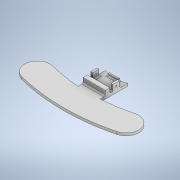
# Autodesk Inventor part: paddle
Saved by Autodesk Inventor 2020.3 (Build 243373010, 373A)
## iProperties
Created: 2020-09-18
Part Number: paddle
Material: Generic
Document SubType Name: Modeling
Designer: joesp
Density: 1 g/cm^3
Appearance: Default
Author: joesp
Autodesk Inventor part; units mm, degrees
ref_plane "YZ Plane" through (0, 0, 0) normal (1, 0, 0) x (0, 1, 0)
ref_plane "XZ Plane" through (0, 0, 0) normal (0, 1, 0) x (-1, 0, 0)
ref_plane "XY Plane" through (0, 0, 0) normal (0, 0, 1) x (1, 0, 0)
sketch "Sketch1" plane through (0, 0, 0) normal (0, 1, 0) x (-1, 0, 0)
  arc A0 (92.5, 31.0634) -> (-57.5, 31.0634) centre (17.5, -259.4104) ccw
  arc A1 (82.5, -7.6665) -> (92.5, 31.0634) centre (87.5, 11.6984) ccw
  arc A2 (-57.5, 31.0634) -> (-47.5, -7.6665) centre (-52.5, 11.6984) ccw
  arc A3 (82.5, -7.6665) -> (-47.5, -7.6665) centre (17.5, -259.4104) ccw
  line L0 (35, 0) -> (0, 0)
  line L1 (0, 0) -> (0, -50)
  line L2 (0, -50) -> (35, -50)
  line L3 (35, -50) -> (35, 0)
  point P0 (40, -0.7704)
  dimension "d0" = 140
  dimension "d1" = 20
  dimension "d2" = 52.5
  dimension "d4" = 300
  dimension "d5" = 50
  dimension "d8" = 35
  dimension "d9" = 52.5
  constraints: 10 point on circle, 8 end point, 4 centre point, 4 tangent, 2 coincident, 2 horizontal alignment, 2 perpendicular, 1 parallel
  measures "d0" distance of A2.centre A1.centre
  measures "d1" radius of A1
  measures "d2" horizontal distance of A1.centre L0.start
  measures "d4" radius of A0
  measures "d5" distance of L2.end L0.start
  measures "d8" distance of L1.end L2.end
  measures "d9" horizontal distance of A2.centre point (0, 0)
extrude "Extrusion1" add sketch "Sketch1" along normal blind 4
sketch "Sketch2" plane through (0, 4, 0) normal (0, 1, 0) x (1, 0, 0)
  line L0 (0, 30) -> (-3, 30)
  line L1 (-3, 30) -> (-3, 20)
  line L2 (-3, 20) -> (0, 20)
  line L3 (0, 20) -> (0, 30)
  line L4 (-35, 30) -> (-32, 30)
  line L5 (-32, 30) -> (-32, 20)
  line L6 (-32, 20) -> (-35, 20)
  line L7 (-35, 20) -> (-35, 30)
  line L8 (0, 0) -> (0, 50) projected
  line L9 (-35, 50) -> (-35, 0) projected
  point P0 (-35, 25)
  dimension "d10" = 3
  dimension "d11" = 3
  dimension "d12" = 10
  constraints: 16 end point, 4 parallel, 2 collinear, 2 horizontal, 2 midpoint, 2 perpendicular, 2 point on line
  measures "d10" distance of L0.start L0.end
  measures "d11" distance of L4.start L4.end
  measures "d12" distance of L4.end L5.end
extrude "Extrusion2" add sketch "Sketch2" along normal blind 10
sketch "Sketch3" plane through (0, 4, 0) normal (0, 1, 0) x (1, 0, 0)
  line L0 (-35, 15) -> (0, 15)
  line L1 (0, 15) -> (0, 8)
  line L2 (0, 8) -> (-35, 8)
  line L3 (-35, 8) -> (-35, 15)
  line L4 (0, 0) -> (0, 20) projected
  line L5 (-35, 20) -> (-35, 0) projected
  line L6 (-35, 50) -> (-35, 0) projected
  point P0 (-35, 25)
  dimension "d15" = 7
  dimension "d16" = 10
  constraints: 8 end point, 2 parallel, 2 point on line, 1 horizontal, 1 midpoint, 1 perpendicular
  measures "d15" distance of L2.end L0.start
  measures "d16" distance from line of L0 point (-35, 25)
extrude "Extrusion3" add sketch "Sketch3" along normal blind 8
sketch "Sketch4" plane through (0, 0, 0) normal (1, 0, 0) x (0, 0, -1)
  circle A0 centre (25, 9) radius 1.375
  line L0 (30, 4) -> (30, 14) projected
  line L1 (20, 14) -> (30, 14) projected
  point P0 (0, 0)
  point P1 (30, 9)
  point P2 (25, 14)
  dimension "d19" = 2.75
  constraints: 2 midpoint, 1 centre point, 1 horizontal alignment, 1 vertical alignment
  measures "d19" diameter of A0
extrude "Extrusion4" cut sketch "Sketch4" against normal through all
sketch "Sketch5" plane through (0, 4, 0) normal (0, 1, 0) x (1, 0, 0)
  line L0 (-25, 37.5) -> (-10, 37.5)
  line L1 (-10, 37.5) -> (-10, 41.5)
  line L2 (-10, 41.5) -> (-25, 41.5)
  line L3 (-25, 41.5) -> (-25, 37.5)
  line L4 (0, 20) -> (0, 30) projected
  line L5 (-35, 50) -> (-35, 30) projected
  line L6 (0, 30) -> (0, 50) projected
  point P0 (0, 0)
  point P1 (-10, 39.5)
  point P2 (0, 25)
  dimension "d22" = 4
  dimension "d23" = 15
  dimension "d26" = 14.5
  dimension "d27" = 10
  dimension "d28" = 10
  constraints: 8 end point, 2 midpoint, 2 parallel, 1 horizontal, 1 perpendicular
  measures "d22" distance of L2.end L0.start
  measures "d23" distance of L0.start L0.end
  measures "d26" vertical distance of point (0, 25) point (-10, 39.5)
  measures "d27" distance between parallel lines of L5 L3
  measures "d28" distance between parallel lines of L6 L1
extrude "Extrusion5" add sketch "Sketch5" along normal blind 3.625
chamfer "Chamfer1" distance 2 angle 45 12 edges at (-17.5, 4, -15) (-32, 4, -25) (-33.5, 4, -30) (-33.5, 4, -20) (-17.5, 4, -8) (-3, 4, -25) (-1.5, 4, -30) (-1.5, 4, -20) (-10, 4, -39.5) (-17.5, 4, -41.5) (-17.5, 4, -37.5) (-25, 4, -39.5)
sketch "Sketch6" plane through (0, 4, 0) normal (0, 1, 0) x (1, 0, 0)
  circle A0 centre (-17.5, 81.5) radius 42
  line L0 (0, 0) -> (0, 50) projected
  line L1 (0, 50) -> (-35, 50) projected
  point P0 (0, 25)
  point P1 (-17.5, 50)
  dimension "d32" = 56.5
  dimension "d33" = 84
  constraints: 2 midpoint, 1 centre point, 1 vertical alignment
  measures "d32" vertical distance of A0.centre point (0, 25)
  measures "d33" diameter of A0
extrude "Extrusion6" cut sketch "Sketch6" along normal through all both and the other way through all
equation "\"d2\" = d9"
equation "\"d11\" = d10"
equation "\"d27\" = d28"
body "Solid1"
